Autodesk Fusion 360 part; units mm, degrees
note: some values were not read from the file. Chosen so that the rebuilt part matches the saved one: which face or edge a step refers to; which pieces of a blend or face edit are solid. Set by a fixed rule: which sketch regions a step uses.
(part 2 of 3)
extrude "Extrude11" cut sketch "Blueprint" along normal blind 2 contours A6 picked at (-1.581142, 47.433122) bodies 1
extrude "Extrude12" add sketch "Blueprint" along normal blind 19 separate body contours L20 L21 L22 L23 A16 A57 | L22 A16 | L22 A56 A57 | L22 A55 A56 | L22 A55 | L3 L7 L24 L26 L27 | L1 A25 picked at (4.033973, -37.441718) picked at (-0.443425, -18.400909) picked at (16, -19.512661) picked at (15.901332, -18.893876) picked at (15.699495, -18.321998) picked at (-6.166027, -29.108385) picked at (17.824648, -25.908449) makes body 3
sketch "Sketch4" plane through (0, 19, 0) normal (0, 1, 0) x (-1, 0, 0)
  line L0 (5.49936, 34.775052) -> (5.49936, 22.275052)
  line L1 (5.49936, 22.275052) -> (-17.60064, 22.275052)
  line L2 (-17.60064, 22.275052) -> (-17.60064, 34.775052)
  line L3 (-17.60064, 34.775052) -> (5.49936, 34.775052)
  line L4 (9.49936, 18.275052) -> (9.49936, 38.775052)
  line L5 (9.49936, 38.775052) -> (-21.60064, 38.775052)
  line L6 (-21.60064, 38.775052) -> (-21.60064, 18.275052)
  line L7 (-21.60064, 18.275052) -> (9.49936, 18.275052)
  line L8 (3.49936, 26.775052) -> (7.49936, 26.775052)
  line L9 (7.49936, 26.775052) -> (7.49936, 30.275052)
  line L10 (7.49936, 30.275052) -> (3.49936, 30.275052)
  line L11 (3.49936, 30.275052) -> (3.49936, 26.775052)
  line L12 (3.49936, 26.775052) -> (7.49936, 30.275052) construction
  line L13 (7.49936, 26.775052) -> (3.49936, 30.275052) construction
  point P0 (5.49936, 28.525052)
  dimension "d49" = 4
  dimension "d50" = 3.5
  constraint horizontal L8
  constraint perpendicular L8 L9
  constraint parallel L8 L10
  constraint parallel L9 L11
extrude "Extrude13" cut sketch "Sketch4" against normal blind 17 contours L0 L8 L9 L10 picked at (6.166027, 29.108385) bodies 3
sketch "Sketch5" plane through (-9.49936, 0, 0) normal (-1, 0, 0) x (0, -1, 0)
  line L0 (0, 18.275052) -> (0, 38.775052)
  line L1 (0, 38.775052) -> (-19, 38.775052)
  line L2 (-19, 38.775052) -> (-19, 18.275052)
  line L3 (-19, 18.275052) -> (0, 18.275052)
  line L4 (-2, 25) -> (-15.110279, 25)
  line L5 (-15.110279, 25) -> (-15.110279, 32.050103)
  line L6 (-15.110279, 32.050103) -> (-2, 32.050103)
  line L7 (-2, 32.050103) -> (-2, 25)
  line L8 (-2, 25) -> (-15.110279, 32.050103) construction
  line L9 (-15.110279, 25) -> (-2, 32.050103) construction
  point P0 (-8.555139, 28.525052)
  constraint horizontal L4
  constraint perpendicular L4 L5
  constraint parallel L4 L6
  constraint parallel L5 L7
extrude "Extrude14" cut sketch "Sketch5" against normal blind 5 contours L4 L5 L6 L7 picked at (-6.370093, 27.350035) bodies 3
extrude "Extrude15" add sketch "Shell" along normal blind 45 separate body makes body 4
extrude "Extrude16" add sketch "Blueprint" along normal blind 45 separate body contours L9 L10 L11 A5 picked at (-1.233383, 60.560963) makes body 5
extrude "Extrude17" add sketch "Shell" along normal blind 2 separate body contours A0 picked at (6.427646, -1.832679) makes body 6
ref_plane "WorkPlane2" through (6.05064, 26, 28.525052) normal (0, 1, 0) x (0, 0, 1)
box "BoxPrimitive1" cut length 17 width 50 height 12 placed x (0, 0, -1) y (-1, 0, 0) z (0, 1, 0) at (25.050639, 26, 61.525052) bodies 4
extrude "Extrude19" add sketch "Blueprint" along normal blind 45 separate body contours A7 | A13 | A23 picked at (-25.103811, -35.273245) picked at (-26.11169, -34.534513) picked at (-29.306987, -35.12917) makes body 7
extrude "Extrude20" add sketch "Blueprint" along normal blind 45 separate body contours A8 | A14 | A22 picked at (-25.103811, 34.726755) picked at (-26.063404, 34.821149) picked at (-29.306987, 34.87083) makes body 8
extrude "Extrude21" add sketch "Blueprint" along normal blind 45 separate body contours A9 | A15 | A21 picked at (25.426628, 33.642904) picked at (29.802492, 35.730779) picked at (27.55602, 33.763856) makes body 9
sketch "Sketch7" plane through (0, 26, 0) normal (0, 1, 0) x (-1, 0, 0)
  arc A0 (24.949361, 47.984679) -> (-25.050639, 47.931884) centre (0, 0) ccw
  line L0 (24.949361, 47.984679) -> (24.949361, 50.228104)
  arc A1 (24.949361, 50.228104) -> (-25.050639, 50.17767) centre (0, 0) ccw
  line L1 (-25.050639, 50.17767) -> (-25.050639, 47.931884)
  circle A2 centre (-19.009017, 51.46438) radius 0.8
  circle A3 centre (-12.981322, 53.323346) radius 0.8
  circle A4 centre (-7.269836, 54.399657) radius 0.8
  circle A5 centre (-1.067304, 54.883088) radius 0.8
  circle A6 centre (4.965873, 54.658118) radius 0.8
  circle A7 centre (10.837016, 53.802717) radius 0.8
  circle A8 centre (16.195064, 52.439423) radius 0.8
  circle A9 centre (21.159709, 50.6403) radius 0.8
  dimension "d80" = 1.6
  dimension "d81" = 1.6
  dimension "d82" = 1.6
  dimension "d83" = 1.6
  dimension "d84" = 1.6
  dimension "d85" = 1.6
  dimension "d86" = 1.6
  dimension "d87" = 1.6
  measures "d80" diameter of A2
  measures "d81" diameter of A3
  measures "d82" diameter of A4
  measures "d83" diameter of A5
  measures "d84" diameter of A6
  measures "d85" diameter of A7
  measures "d86" diameter of A8
  measures "d87" diameter of A9
extrude "Extrude22" add sketch "Sketch7" along normal blind 12 contours A0 A2 picked at (-18.916947, 51.228603) bodies 4
extrude "Extrude23" add sketch "Sketch7" along normal blind 12 contours A0 A3 picked at (-13.069534, 53.575351) bodies 4
extrude "Extrude24" add sketch "Sketch7" along normal blind 12 contours A4 picked at (-6.832624, 54.634154) bodies 4
extrude "Extrude25" add sketch "Sketch7" along normal blind 12 contours A5 picked at (-0.753146, 55.064467) bodies 4
extrude "Extrude26" add sketch "Sketch7" along normal blind 12 contours A6 picked at (5.19146, 54.520452) bodies 4
extrude "Extrude27" add sketch "Sketch7" along normal blind 12 contours A7 picked at (11.203399, 54.016143) bodies 4
extrude "Extrude28" add sketch "Sketch7" along normal blind 12 contours A8 picked at (15.936855, 52.760909) bodies 4
extrude "Extrude29" add sketch "Sketch7" along normal blind 12 contours A9 picked at (21.418616, 50.832786) bodies 4
delete_face "DeleteFace1" 2 faces at (-21.958832, 34, 50.602854) (-20.364995, 34, 50.732108) on bodies 4
delete_face "DeleteFace2" 1 faces at (-15.399192, 34, 52.520588) on bodies 4
delete_face "DeleteFace3" 1 faces at (-11.633153, 34, 53.724196) on bodies 4
delete_face "DeleteFace4" 1 faces at (-4.169017, 34, 54.587261) on bodies 4
delete_face "DeleteFace5" 1 faces at (1.769881, 34, 54.500485) on bodies 4
delete_face "DeleteFace6" 1 faces at (8.044162, 34, 54.600699) on bodies 4
delete_face "DeleteFace7" 1 faces at (13.706571, 30, 52.985687) on bodies 4
delete_face "DeleteFace8" 1 faces at (19.672072, 34, 51.911994) on bodies 4
extrude "Extrude30" cut sketch "Blueprint" along normal blind 2 contours A2 | A10 | A11 | A24 picked at (28.037278, -34.616147) picked at (26.387387, -34.993527) picked at (26.938574, -33.213382) picked at (27.869684, -36.306977) bodies 6
extrude "Extrude31" add sketch "Blueprint" along normal blind 40 separate body contours A12 picked at (26.253933, -32.672943) makes body 10
extrude "Extrude32" add 1 faces at (-42.36532, 0, -35.508369) along direction (0, 1, 0) blind 3 from surface at 45 separate body on bodies 4 makes body 11
extrude "Extrude33" add 1 faces at (-1.233383, 45, -60.560963) along direction (0, 1, 0) blind 5 separate body on bodies 5 makes body 12
extrude "Extrude34" add 1 faces at (-42.36532, 0, -35.508369) along direction (0, 1, 0) blind 5 from surface at 45 separate body on bodies 4 makes body 13
extrude "Extrude35" add sketch "Blueprint" against normal blind 2 from surface at 50 separate body contours A0 L454 | A0 L40 L46 A46 L497 | A0 L40 L46 L454 | A0 A46 L497 L498 | A0 L40 L46 A46 L498 | A0 L32 L40 L46 A46 | A0 L32 L40 L46 | A16 L40 L46 A46 L497 | A16 A46 L497 L498 L499 | A0 L32 L40 L46 A46 | A16 L40 L46 A46 L498 L499 | L32 A16 L40 L46 A46 | L30 L31 L33 A16 L40 L46 A33 L423 L428 L429 L437 L440 L441 L449 A43 L455 L456 L457 L490 L491 L494 L495 A49 | A0 L32 L38 | A0 L32 L38 A46 | L32 A16 L40 L46 A46 | A0 L32 L38 A46 | L32 A16 L40 L43 L46 L49 L459 L462 L479 L480 L481 L484 L485 L489 L490 | A0 L38 L48 | A0 L38 L48 A46 | L32 L38 A16 A46 | L32 A16 L40 L41 L46 L47 L397 L400 L401 L407 L408 L411 L415 L416 L423 | A0 L38 L48 A46 | L32 L38 A16 A46 | L33 L40 L43 L46 L49 L489 L490 L491 | L40 L43 L46 L49 L489 L490 | A0 L42 L48 | A0 L42 L48 A46 | L38 A16 L48 A46 | L32 L38 A16 L397 | L40 L41 L46 L47 L416 L423 | L31 L40 L41 L46 L47 L416 L423 L428 | A0 L42 L48 A46 | L38 A16 L48 A46 | L32 L38 A16 L462 | A0 L42 | A0 L42 A46 | A16 L42 L48 A46 | L38 A16 L48 L397 | L32 L38 L41 L47 L397 | L32 L41 L47 L397 L400 | A16 L42 L48 A46 | L38 A16 L48 L462 | L32 L43 L49 L459 L462 | L32 L38 L43 L49 L462 | L33 L43 L49 L481 L489 | L33 L39 L345 L346 L347 L489 L491 | L33 L39 L455 L491 | L22 A16 L42 A46 | A16 L42 L48 L397 | L38 L41 L47 L48 L397 | L31 L32 L37 L38 L41 L47 L396 L399 L400 | L31 L32 L41 L47 L400 | L31 L41 L47 L415 L416 | L31 L37 L428 L429 | L31 L37 L416 L419 L420 L427 L428 | A16 L42 L48 L462 | L38 L43 L48 L49 L462 | L32 L33 L43 L49 L459 | L32 L33 L38 L39 L43 L49 L342 L343 L459 | L33 L43 L49 L481 L484 | L43 L49 L479 L480 L481 L484 L485 | L33 L39 L481 L489 | L33 L455 L456 L457 | L33 L39 L320 L321 L322 L455 L457 | L39 L315 L347 L491 | L39 L315 L455 L491 | L41 L42 L48 L397 | L37 L38 L41 L42 L47 L389 L390 L391 L393 L396 L397 L399 L400 | L31 L41 L47 L400 L401 | L41 L47 L401 L407 L408 L411 L415 | L31 L41 L47 L401 L415 | L31 L37 L415 L416 | L31 L37 L429 L431 L436 L439 L440 | L31 L429 L437 L440 | L37 L416 L418 L419 L425 L427 L428 | L42 L43 L48 L462 | L38 L42 L43 L49 L315 L341 L342 L461 L462 | L33 L43 L49 L459 L484 | L33 L39 L324 L325 L326 L481 L484 | L39 L315 L481 L489 | L39 L315 L345 L489 | L33 L39 L457 L494 | L39 L315 L320 L455 | L39 L220 L313 L315 L347 | L39 L219 L220 L265 L281 L287 L313 L345 L346 L347 | L315 L345 L347 L348 L489 L491 L492 | L20 L21 L22 L23 A16 A57 | L22 A16 | L37 L38 L391 L392 L393 L394 L395 L396 L398 L399 | L37 L38 L395 L396 L398 L399 | L31 L37 L400 L401 | L31 L37 L401 L404 L406 L414 L415 | L31 L37 L440 L441 | L37 L429 L430 L431 L432 L439 L440 | L37 L419 L420 L421 L422 L426 L427 | L37 L419 L422 L424 L425 L426 L427 | L38 L39 L227 L247 L251 L295 L342 L343 | L38 L227 L249 L251 L303 L315 L341 L342 | L33 L39 L459 L484 | L39 L315 L326 L481 | L39 L265 L281 L315 L345 | L30 L33 L494 L495 | L30 L33 L36 L39 L349 L350 L494 L495 | L39 L315 L322 L457 | L39 L315 L457 L494 | L39 L218 L222 L228 L284 L293 L298 L320 L321 L322 | L39 L218 L284 L315 L320 | L315 L320 L322 L323 L455 L457 L458 | L39 L220 L265 L281 L313 L315 | L39 L219 L220 L265 L281 L287 L313 | L220 L265 L266 L273 L281 L313 L315 L345 L347 L348 | L37 L38 L392 L394 L395 L398 | L37 L38 L395 L398 | L37 L401 L402 L403 L404 L412 L414 L415 L417 | L30 L31 L36 L37 L441 L443 L448 L449 | L30 L31 L441 L449 | L37 L431 L432 L433 L434 L438 L439 | L37 L431 L433 L435 L436 L438 L439 | L37 L421 L422 L426 | L37 L422 L424 L426 | L22 A56 A57 | L22 A56 A57 | L38 L39 L227 L247 L251 L295 | L38 L39 L227 L247 L249 L251 L295 L303 L315 | L39 L315 L343 L459 | L39 L315 L459 L484 | L39 L315 L324 L484 | L39 L271 L314 L315 L326 | L39 L216 L231 L252 L267 L271 L314 L324 L325 L326 | L315 L324 L326 L327 L478 L481 L482 L483 L484 | L39 L315 L349 L494 | L39 L222 L228 L315 L322 | L39 L218 L222 L228 L284 L293 L298 | L39 L218 L222 L228 L284 L315 | L218 L222 L228 L237 L240 L284 L315 L320 L322 L323 | L220 L265 L266 L273 L281 L313 L315 | L37 L404 L405 L406 L409 L413 L414 | L37 L403 L404 L409 L410 L413 L414 | L36 L37 L441 L442 L443 L444 L448 L449 L451 L452 | L37 L433 L434 L438 | L37 L433 L435 L438 | L22 A55 A56 | L22 A55 A56 | L315 L341 L343 L344 L459 L460 L461 | L236 L242 L247 L249 L295 L303 L315 L341 L343 L344 | L39 L247 L295 L315 L343 | L39 L231 L252 L315 L324 | L39 L231 L252 L271 L314 L315 | L39 L216 L231 L252 L267 L271 L314 | L231 L252 L268 L271 L275 L314 L315 L324 L326 L327 | L30 L36 A33 L495 | L36 L39 L229 L254 L299 L309 L349 L350 | L39 L229 L254 L315 L349 | L315 L349 L351 L352 L493 L494 L496 | L218 L222 L228 L237 L240 L284 L315 | L37 L405 L409 L413 | L37 L409 L410 L413 | L30 L36 L449 A43 | L36 L37 L443 L444 L445 L446 L447 L448 L450 L451 | L36 L37 L443 L446 L447 L448 | L22 A55 | L22 A55 | L236 L242 L247 L249 L295 L303 L315 | L231 L252 L268 L271 L275 L314 L315 | L30 A32 A33 | L30 L36 A32 A33 | L36 L315 L350 L351 L495 L496 | L36 L39 L229 L254 L299 L309 | L36 L39 L223 L229 L254 L292 L299 L309 L315 | L223 L229 L234 L241 L254 L292 L315 L349 L351 L352 | L30 L36 A43 A44 | L30 A43 A44 | L36 L37 L445 L446 L447 L450 | L36 L37 L446 L447 | L30 A31 A32 | L30 L36 A31 A32 | L30 L36 A32 A33 | L30 L36 A33 A49 | L36 A32 A33 | L36 L223 L292 L299 L309 L315 L350 L351 | L223 L229 L234 L241 L254 L292 L315 | L30 L36 A44 A45 | L30 A44 A45 | L36 A43 A44 | L30 L36 A43 A49 | L30 L36 A43 A44 | L30 A31 | L30 L36 A31 | L30 L36 A31 A32 | L36 A31 A32 | L30 A49 A51 | L30 L36 A49 A51 | L30 L36 A45 | L30 A45 | L36 A44 A45 | L30 L36 A44 A45 | L30 L36 A49 A51 | L36 A31 | L30 A50 A51 | L30 L36 A50 A51 | L36 A49 A51 | L36 A45 | L30 L36 A50 A51 | L30 A50 | L30 L36 A50 | L36 A50 A51 | L36 A50 | L0 L2 L3 L4 L5 L6 L7 L24 L25 L26 | L0 L1 L2 L5 A25 | L3 L7 L24 L26 L27 | L3 L7 L24 L25 L26 | L1 A25 | L1 A25 | L8 L9 L11 A5 | L8 L9 L11 L14 L15 L17 A5 | L14 L15 L17 A5 | A1 | A2 | A3 | A4 | A6 | A7 | A8 | A9 | A10 | A11 | A12 | A13 | A14 | A15 | A17 | A18 | A19 | A21 | A22 | A23 | A24 | L235 L260 L270 L286 L288 L301 L315 L328 L329 L331 | L235 L260 L270 L286 L288 L301 L315 | L246 L259 L260 L286 L288 L301 L315 | L246 L259 L260 L286 L288 L301 L315 L329 L330 L331 | L315 L329 L330 L331 L471 L472 L473 | L315 L328 L329 L331 L471 L473 L474 | L238 L243 L244 L248 L264 L307 L315 L332 L334 L335 | L238 L243 L244 L248 L264 L307 L315 | L244 L248 L264 L279 L300 L307 L315 | L244 L248 L264 L279 L300 L307 L315 L332 L333 L334 | L315 L332 L333 L334 L464 L465 L466 | L315 L332 L334 L335 L463 L464 L466 | L239 L245 L272 L278 L290 L297 L315 L336 L338 L339 | L239 L245 L272 L278 L290 L297 L315 | L245 L261 L278 L289 L290 L297 L315 | L245 L261 L278 L289 L290 L297 L315 L336 L337 L338 | L315 L336 L337 L338 L467 L468 L470 | L315 L336 L338 L339 L468 L469 L470 | A26 | A27 | A28 | A29 | A30 | A34 | A35 | A36 | A37 | A38 | A39 | L353 L354 L355 L356 | L357 L360 L362 L363 | L358 L359 L361 L364 | L365 L366 L367 L376 | L368 L371 L373 L375 | L369 L370 L372 L374 | L377 L378 L379 L388 | L380 L383 L385 L387 | L381 L382 L384 L386 | A40 | A41 | A42 | A52 | A53 | A54 picked at (-0.080266, 16.579553) picked at (9.705176, 15.068275) picked at (-3, 10.157626) picked at (-7.671277, 16.192817) picked at (-9.705176, 15.068275) picked at (16.610892, 6.696031) picked at (5.417667, 1.4) picked at (10.29341, 15.063896) picked at (8.168486, 16.306197) picked at (-16.588449, 6.769971) picked at (-10.29341, 15.063896) picked at (16.955543, 6.695503) picked at (-18.919314, 15.014678) picked at (-5.900918, -1.983333) picked at (-17.768839, -2.539148) picked at (-16.933326, 6.769391) picked at (17.768839, -2.539148) picked at (22.633332, 0.538942) picked at (-5.882271, -2.766667) picked at (-17.703996, -2.961152) picked at (-18.088769, -2.539143) picked at (-22.551552, 3.200808) picked at (17.703996, -2.961152) picked at (18.088769, -2.539143) picked at (24.886666, 10.733333) picked at (24.733332, 6.85) picked at (5.683555, -5.514289) picked at (-16.506733, -7.014289) picked at (-18.061761, -2.727855) picked at (-22.598153, -2.094669) picked at (-24.866667, 6.85) picked at (-24.886667, 10.733333) picked at (16.506733, -7.014289) picked at (18.061761, -2.727855) picked at (22.59815, -2.094669) picked at (-1.266033, -11.46973) picked at (15.487236, -8.996433) picked at (-16.85228, -7.014027) picked at (-22.570428, -2.766667) picked at (-24.866667, -1.983333) picked at (-24.733335, -1.583333) picked at (16.85228, -7.014027) picked at (22.570425, -2.766667) picked at (24.733332, -1.516667) picked at (24.733332, -1.983333) picked at (25.04, 5.483333) picked at (25.489999, 12.1) picked at (25.393333, 12.416666) picked at (-3.872417, -17.820116) picked at (-22.447225, -5.011798) picked at (-24.866667, -2.766667) picked at (-25.490001, -1.766667) picked at (-25.02, -1.583333) picked at (-25.02, 5.483333) picked at (-25.393333, 12.383333) picked at (-25.490001, 12.1) picked at (22.447222, -5.011798) picked at (24.866666, -2.883333) picked at (25.04, -1.583333) picked at (25.489999, -1.766667) picked at (25.02, 3.183333) picked at (24.866666, 2.355609) picked at (25.726667, 5.483333) picked at (24.906666, 14.716666) picked at (25.489999, 12.7) picked at (27.353333, 11.85) picked at (27.353333, 12.383333) picked at (-24.866667, -4.5) picked at (-28.883336, -8) picked at (-25.02, -1.416667) picked at (-24.866667, 1.744392) picked at (-25.04, 3.183333) picked at (-25.726667, 5.516666) picked at (-25.490001, 19) picked at (-24.906667, 16.983333) picked at (-31.150002, 9.833333) picked at (24.733332, -4.5) picked at (25.983332, -8) picked at (25.02, -1.383334) picked at (25.489999, -1.1) picked at (27.353333, 5.483333) picked at (27.353333, 5.8) picked at (25.393333, 19.316666) picked at (27.353333, 12.7) picked at (27.353333, 11.5) picked at (25.399998, 8.116666) picked at (31.149998, 8.066666) picked at (4.033973, -37.441718) picked at (-0.443425, -18.400909) picked at (-27.166669, -7.45) picked at (-25.636668, -2.25) picked at (-25.726667, -1.383334) picked at (-25.490001, -1.1) picked at (-25.393333, 19.283333) picked at (-31.150002, 14.966666) picked at (-25.400002, 8.116666) picked at (-30.600002, 8.116666) picked at (25.636665, -2.25) picked at (25.399998, -5.833333) picked at (25.393333, -1.383334) picked at (27.353333, 4.95) picked at (27.353333, 6.35) picked at (24.906666, 20.116667) picked at (25.489999, 19.6) picked at (27.353333, 18.75) picked at (27.353333, 19.283333) picked at (25.399998, 16.683333) picked at (27.353333, 13.25) picked at (31.149998, 14.966666) picked at (27.353333, 8.116666) picked at (25.873333, 8.116666) picked at (30.599998, 8.116666) picked at (-27.353335, -5.783333) picked at (-25.873334, -2.45) picked at (-30.900002, 2.355609) picked at (-25.490001, 19.6) picked at (-24.906667, 20.883333) picked at (-30.600002, 16.683333) picked at (-25.400002, 15.016666) picked at (-25.873334, 9.783333) picked at (-29.020002, 9.783333) picked at (14.100388, -18.043793) picked at (16, -19.512661) picked at (25.686665, -2.45) picked at (26.519999, -5.783333) picked at (27.353333, -1.95) picked at (27.353333, -1.416667) picked at (27.353333, -1.1) picked at (27.353333, 4.6) picked at (25.399998, 1.216666) picked at (30.899998, 1.744392) picked at (27.353333, 19.6) picked at (27.353333, 18.4) picked at (25.873333, 15.016666) picked at (27.353333, 15.016666) picked at (30.599998, 15.016666) picked at (28.833332, 9.783333) picked at (-25.400002, 1.216666) picked at (-30.600002, 1.216666) picked at (-31.150002, 21.866666) picked at (-27.540001, 15.016666) picked at (-25.873334, 16.683333) picked at (14.799711, -18.162342) picked at (15.901332, -18.893876) picked at (31.149998, -5.733334) picked at (30.599998, -4.016667) picked at (27.353333, -2.3) picked at (27.353333, -0.55) picked at (27.353333, 1.216666) picked at (25.686665, 2.883333) picked at (30.599998, 2.883333) picked at (22.473627, 22.229735) picked at (25.399998, 21) picked at (27.353333, 20.15) picked at (31.149998, 21.866666) picked at (28.833332, 16.683333) picked at (-25.873334, 2.883333) picked at (-29.020002, 2.883333) picked at (-22.806963, 22.229735) picked at (-27.166669, 25.35) picked at (-25.400002, 21) picked at (15.900371, -17.570903) picked at (15.699495, -18.321998) picked at (28.833333, -4.016667) picked at (28.833333, 2.883333) picked at (14.739817, 21.245372) picked at (17.917968, 22.326792) picked at (24.849998, 24.733333) picked at (25.873333, 21.05) picked at (27.353333, 22.716667) picked at (30.599998, 21.916666) picked at (-18.917967, 22.326792) picked at (-18.260183, 21.245372) picked at (-29.020002, 22.716667) picked at (-25.873334, 21.85) picked at (15.401746, 21.543061) picked at (16.918149, 21.76373) picked at (14.082033, 22.326792) picked at (6.082593, 22.476137) picked at (14.039145, 22.826574) picked at (25.399998, 24.433333) picked at (28.833332, 23.583333) picked at (-17.918148, 21.76373) picked at (-16.401745, 21.543061) picked at (-18.960855, 22.826574) picked at (-6.415925, 22.476137) picked at (-15.082032, 22.326792) picked at (16.144253, 21.625767) picked at (15.793173, 22.25812) picked at (15.081852, 21.76373) picked at (14.653406, 22.779056) picked at (-1.260183, 21.245372) picked at (1.917968, 22.326792) picked at (-16.76103, 22.289882) picked at (-16.855747, 21.625767) picked at (-18.346594, 22.779056) picked at (-16.081851, 21.76373) picked at (-1.917967, 22.326792) picked at (16.399841, 22.897923) picked at (-0.598254, 21.543061) picked at (0.918149, 21.76373) picked at (-1.960855, 22.826574) picked at (-16.838019, 23.067226) picked at (-0.918148, 21.76373) picked at (-0.144252, 21.625767) picked at (0.269322, 21.884696) picked at (-1.346594, 22.779056) picked at (0.161981, 23.067226) picked at (-1.166027, -27.941718) picked at (4.61622, -27.751627) picked at (-6.166027, -29.108385) picked at (-4.832694, -27.941718) picked at (17.274712, -27.041797) picked at (17.824648, -25.908449) picked at (-19.500414, 45.97393) picked at (-0.092673, 33.048676) picked at (1.364052, -47.916694) picked at (-28.447805, -34.584499) picked at (28.037278, -34.616147) picked at (27.665869, 35.49322) picked at (-28.447805, 35.415501) picked at (-1.581142, 47.433122) picked at (-25.103811, -35.273245) picked at (-25.103811, 34.726755) picked at (25.426628, 33.642904) picked at (26.387387, -34.993527) picked at (26.938574, -33.213382) picked at (26.253933, -32.672943) picked at (-26.11169, -34.534513) picked at (-26.063404, 34.821149) picked at (29.802492, 35.730779) picked at (38.740213, -25.999966) picked at (39.611389, -23.686242) picked at (37.680599, -25.819207) picked at (27.55602, 33.763856) picked at (-29.306987, 34.87083) picked at (-29.306987, -35.12917) picked at (27.869684, -36.306977) picked at (30.599998, -10.916667) picked at (28.833333, -10.916667) picked at (27.166666, -12.583334) picked at (25.399998, -12.583334) picked at (24.849998, -12.633334) picked at (31.149998, -12.633334) picked at (30.599998, -17.816667) picked at (28.833333, -17.816667) picked at (27.166666, -19.483334) picked at (25.399998, -19.483334) picked at (24.849998, -17.766667) picked at (31.149998, -19.533334) picked at (30.599998, -24.716667) picked at (28.833333, -24.716667) picked at (27.166666, -26.383334) picked at (25.399998, -26.383334) picked at (24.849998, -24.666667) picked at (31.149998, -26.433334) picked at (16.330409, -25.375998) picked at (17.340134, -25.681655) picked at (39.344267, 22.860514) picked at (39.611389, 24.613758) picked at (37.680599, 22.480793) picked at (-39.655733, -25.439486) picked at (-41.319401, -25.819207) picked at (-39.388611, -23.686242) picked at (-15.04171, -25.661782) picked at (-15.655212, -25.619554) picked at (-16.643107, -25.607971) picked at (-31.150002, -24.666667) picked at (-25.400002, -26.383334) picked at (-28.833336, -24.716667) picked at (-31.150002, -17.766667) picked at (-27.166669, -21.25) picked at (-27.166669, -19.483334) picked at (-28.883336, -14.9) picked at (-25.400002, -10.916667) picked at (-27.166669, -12.583334) picked at (-41.319401, 22.480793) picked at (-39.655733, 22.860514) picked at (-39.388611, 24.613758) picked at (-16.643107, -17.607971) picked at (-15.655212, -17.619554) picked at (-15.046922, -17.731335) makes body 14
sketch "Sketch8" plane through (0, 48, 0) normal (0, 1, 0) x (-1, 0, 0)
  circle A0 centre (0, 0) radius 53.966054
  circle A1 centre (-28, 35.000001) radius 1.25
  circle A2 centre (-28, 35.000001) radius 1.75
  circle A3 centre (-28, 35.000001) radius 2.236068
  circle A4 centre (0, 0) radius 54.966054
  circle A5 centre (-28, 35.000001) radius 3.4
  circle A6 centre (-28, 35.000001) radius 4.9
  circle A7 centre (0, 0) radius 18.05
  circle A8 centre (0, 0) radius 18.7
  line L0 (-9, -15.472879) -> (9, -15.472879)
  line L1 (9.294757, -15.472879) -> (10.501428, -15.472879)
  line L2 (9, -15.472879) -> (10.8, -15.472879)
  line L3 (-9, -15.472879) -> (-11.1, -15.472879)
  circle A9 centre (-16, 17.550001) radius 2.25
  circle A10 centre (-16, 17.550001) radius 1.4
  circle A11 centre (-16, 17.550001) radius 1.25
  circle A12 centre (-16, 25.550001) radius 1.25
  circle A13 centre (-16, 25.550001) radius 1.4
  circle A14 centre (-16, 25.550001) radius 2.25
  circle A15 centre (17, 25.550001) radius 2.25
  circle A16 centre (17, 25.550001) radius 1.25
  circle A17 centre (17, 25.550001) radius 1.4
  circle A18 centre (17, 17.550001) radius 2.25
  circle A19 centre (17, 17.550001) radius 1.4
  circle A20 centre (17, 17.550001) radius 1.25
  circle A21 centre (40, 25.550001) radius 2.25
  circle A22 centre (40, 25.550001) radius 1.25
  circle A23 centre (40, 25.550001) radius 1.4
  circle A24 centre (40, -22.749999) radius 2.25
  circle A25 centre (40, -22.749999) radius 1.4
  circle A26 centre (40, -22.749999) radius 1.25
  circle A27 centre (17, -22.749999) radius 2.25
  circle A28 centre (17, -22.749999) radius 1.4
  circle A29 centre (17, -22.749999) radius 1.25
  circle A30 centre (0, -22.749999) radius 2.25
  circle A31 centre (0, -22.749999) radius 1.4
  circle A32 centre (0, -22.749999) radius 1.25
  circle A33 centre (-16, -22.749999) radius 2.25
  circle A34 centre (-16, -22.749999) radius 1.4
  circle A35 centre (-16, -22.749999) radius 1.25
  circle A36 centre (-39, -22.749999) radius 2.25
  circle A37 centre (-39, -22.749999) radius 1.4
  circle A38 centre (-39, -22.749999) radius 1.25
  circle A39 centre (-39, 25.550001) radius 2.25
  circle A40 centre (-39, 25.550001) radius 1.4
  circle A41 centre (-39, 25.550001) radius 1.25
  line L4 (-30.649998, 28.2) -> (-25.349998, 28.2)
  line L5 (-25.349998, 28.2) -> (-25.349998, 22.9)
  line L6 (-25.349998, 22.9) -> (-30.649998, 22.9)
  line L7 (-30.649998, 22.9) -> (-30.649998, 28.2)
  line L8 (-31.399998, 28.95) -> (-24.599998, 28.95)
  line L9 (-24.599998, 28.95) -> (-24.599998, 22.15)
  line L10 (-24.599998, 22.15) -> (-31.399998, 22.15)
  line L11 (-31.399998, 22.15) -> (-31.399998, 28.95)
  line L12 (-31.399998, 22.05) -> (-24.599998, 22.05)
  line L13 (-24.599998, 22.05) -> (-24.599998, 15.25)
  line L14 (-25.349998, 21.3) -> (-25.349998, 16)
  line L15 (-30.649998, 21.3) -> (-25.349998, 21.3)
  line L16 (-30.649998, 16) -> (-30.649998, 21.3)
  line L17 (-31.399998, 15.25) -> (-31.399998, 22.05)
  line L18 (-25.349998, 16) -> (-30.649998, 16)
  line L19 (-24.599998, 15.25) -> (-31.399998, 15.25)
  line L20 (-24.599998, 15.15) -> (-24.599998, 8.35)
  line L21 (-31.399998, 15.15) -> (-24.599998, 15.15)
  line L22 (-22, 15.200001) -> (-34, 15.200001)
  line L23 (-31.399998, 8.35) -> (-31.399998, 15.15)
  line L24 (-25.349998, 14.4) -> (-25.349998, 9.1)
  line L25 (-30.649998, 14.4) -> (-25.349998, 14.4)
  line L26 (-30.649998, 9.1) -> (-30.649998, 14.4)
  line L27 (-25.349998, 9.1) -> (-30.649998, 9.1)
  line L28 (-24.599998, 8.35) -> (-31.399998, 8.35)
  line L29 (-31.399998, 8.25) -> (-24.599998, 8.25)
  line L30 (-24.599998, 8.25) -> (-24.599998, 1.45)
  line L31 (-30.649998, 7.5) -> (-25.349998, 7.5)
  line L32 (-30.649998, 2.2) -> (-30.649998, 7.5)
  line L33 (-31.399998, 1.45) -> (-31.399998, 8.25)
  line L34 (-25.349998, 7.5) -> (-25.349998, 2.2)
  line L35 (-25.349998, 2.2) -> (-30.649998, 2.2)
  line L36 (-24.599998, 1.45) -> (-31.399998, 1.45)
  line L37 (-31.399998, 1.35) -> (-24.599998, 1.35)
  line L38 (-24.599998, 1.35) -> (-24.599998, -2.966827)
  line L39 (-30.649998, 0.6) -> (-25.349998, 0.6)
  line L40 (-25.349998, 0.6) -> (-25.349998, -4.7)
  line L41 (-30.649998, -4.7) -> (-30.649998, 0.6)
  line L42 (-31.399998, -1.133176) -> (-31.399998, 0.943173)
  line L43 (-31.399998, 0.943173) -> (-31.399998, 1.35)
  line L44 (-31.399998, -5.45) -> (-31.399998, -1.133176)
  line L45 (-24.599998, -2.966827) -> (-24.599998, -5.043176)
  line L46 (-24.599998, -5.043176) -> (-24.599998, -5.45)
  line L47 (-24.599998, -5.45) -> (-31.399998, -5.45)
  line L48 (-24.599998, -5.55) -> (-24.599998, -12.35)
  line L49 (-31.399998, -5.55) -> (-24.599998, -5.55)
  line L50 (-30.649998, -6.3) -> (-25.349998, -6.3)
  line L51 (-30.649998, -11.6) -> (-30.649998, -6.3)
  line L52 (-25.349998, -6.3) -> (-25.349998, -11.6)
  line L53 (-31.399998, -12.35) -> (-31.399998, -5.55)
  line L54 (-25.349998, -11.6) -> (-30.649998, -11.6)
  line L55 (-24.599998, -12.45) -> (-24.599998, -19.25)
  line L56 (-30.649998, -13.2) -> (-25.349998, -13.2)
  line L57 (-24.599998, -12.35) -> (-31.399998, -12.35)
  line L58 (-31.399998, -12.45) -> (-24.599998, -12.45)
  line L59 (-31.399998, -19.25) -> (-31.399998, -12.45)
  line L60 (-30.649998, -18.5) -> (-30.649998, -13.2)
  line L61 (-25.349998, -13.2) -> (-25.349998, -18.5)
  line L62 (-25.349998, -18.5) -> (-30.649998, -18.5)
  line L63 (-31.399998, -19.35) -> (-24.599998, -19.35)
  line L64 (-24.599998, -19.25) -> (-31.399998, -19.25)
  line L65 (-24.599998, -19.35) -> (-24.599998, -26.15)
  line L66 (-31.399998, -26.15) -> (-31.399998, -19.35)
  line L67 (-30.649998, -20.1) -> (-25.349998, -20.1)
  line L68 (-25.349998, -20.1) -> (-25.349998, -25.4)
  line L69 (-30.649998, -25.4) -> (-30.649998, -20.1)
  line L70 (-25.349998, -25.4) -> (-30.649998, -25.4)
  line L71 (-24.599998, -26.15) -> (-31.399998, -26.15)
  line L72 (-25.349998, -4.7) -> (-30.649998, -4.7)
  line L73 (-30.499998, 0.45) -> (-25.499998, 0.45)
  line L74 (-25.499998, 0.45) -> (-25.499998, -4.55)
  line L75 (-30.499998, -4.55) -> (-30.499998, 0.45)
  line L76 (-25.499998, -4.55) -> (-30.499998, -4.55)
  line L77 (25.350002, 28.2) -> (30.650002, 28.2)
  line L78 (25.350002, 22.9) -> (25.350002, 28.2)
  line L79 (24.600002, 22.15) -> (24.600002, 28.95)
  line L80 (24.600002, 28.95) -> (31.400002, 28.95)
  line L81 (31.400002, 28.95) -> (31.400002, 22.15)
  line L82 (30.650002, 28.2) -> (30.650002, 22.9)
  line L83 (31.400002, 22.15) -> (24.600002, 22.15)
  line L84 (30.650002, 22.9) -> (25.350002, 22.9)
  line L85 (24.600002, 22.05) -> (31.400002, 22.05)
  line L86 (24.600002, 15.25) -> (24.600002, 22.05)
  line L87 (25.350002, 21.3) -> (30.650002, 21.3)
  line L88 (25.350002, 16) -> (25.350002, 21.3)
  line L89 (30.650002, 21.3) -> (30.650002, 16)
  line L90 (31.400002, 22.05) -> (31.400002, 15.25)
  line L91 (30.650002, 16) -> (25.350002, 16)
  line L92 (31.400002, 15.25) -> (24.600002, 15.25)
  line L93 (24.600002, 15.15) -> (31.400002, 15.15)
  line L94 (24.600002, 8.35) -> (24.600002, 15.15)
  line L95 (25.350002, 14.4) -> (30.650002, 14.4)
  line L96 (25.350002, 9.1) -> (25.350002, 14.4)
  line L97 (30.650002, 14.4) -> (30.650002, 9.1)
  line L98 (31.400002, 15.15) -> (31.400002, 8.35)
  line L99 (31.400002, 8.35) -> (24.600002, 8.35)
  line L100 (30.650002, 9.1) -> (25.350002, 9.1)
  line L101 (24.600002, 1.45) -> (24.600002, 8.25)
  line L102 (25.350002, 7.5) -> (30.650002, 7.5)
  line L103 (24.600002, 8.25) -> (31.400002, 8.25)
  line L104 (25.350002, 2.2) -> (25.350002, 7.5)
  line L105 (30.650002, 7.5) -> (30.650002, 2.2)
  line L106 (31.400002, 8.25) -> (31.400002, 1.45)
  line L107 (31.400002, 1.45) -> (24.600002, 1.45)
  line L108 (30.650002, 2.2) -> (25.350002, 2.2)
  line L109 (24.600002, 1.35) -> (31.400002, 1.35)
  line L110 (24.600002, 0.943173) -> (24.600002, 1.35)
  line L111 (24.600002, -1.133176) -> (24.600002, 0.943173)
  line L112 (25.350002, 0.6) -> (30.650002, 0.6)
  line L113 (25.350002, -4.7) -> (25.350002, 0.6)
  line L114 (30.650002, 0.6) -> (30.650002, -4.7)
  line L115 (31.400002, 1.35) -> (31.400002, -2.966827)
  line L116 (24.600002, -5.45) -> (24.600002, -1.133176)
  line L117 (30.650002, -4.7) -> (25.350002, -4.7)
  line L118 (31.400002, -2.966827) -> (31.400002, -5.043176)
  line L119 (31.400002, -5.043176) -> (31.400002, -5.45)
  line L120 (31.400002, -5.45) -> (24.600002, -5.45)
  line L121 (24.600002, -12.35) -> (24.600002, -5.55)
  line L122 (24.600002, -5.55) -> (31.400002, -5.55)
  line L123 (25.350002, -6.3) -> (30.650002, -6.3)
  line L124 (25.350002, -11.6) -> (25.350002, -6.3)
  line L125 (30.650002, -6.3) -> (30.650002, -11.6)
  line L126 (31.400002, -5.55) -> (31.400002, -12.35)
  line L127 (30.650002, -11.6) -> (25.350002, -11.6)
  line L128 (31.400002, -12.35) -> (24.600002, -12.35)
  line L129 (24.600002, -12.45) -> (31.400002, -12.45)
  line L130 (24.600002, -19.25) -> (24.600002, -12.45)
  line L131 (25.350002, -13.2) -> (30.650002, -13.2)
  line L132 (25.350002, -18.5) -> (25.350002, -13.2)
  line L133 (30.650002, -13.2) -> (30.650002, -18.5)
  line L134 (31.400002, -12.45) -> (31.400002, -19.25)
  line L135 (30.650002, -18.5) -> (25.350002, -18.5)
  line L136 (31.400002, -19.25) -> (24.600002, -19.25)
  line L137 (24.600002, -19.35) -> (31.400002, -19.35)
  line L138 (24.600002, -26.15) -> (24.600002, -19.35)
  line L139 (25.350002, -20.1) -> (30.650002, -20.1)
  line L140 (30.650002, -20.1) -> (30.650002, -25.4)
  line L141 (31.400002, -19.35) -> (31.400002, -26.15)
  line L142 (25.350002, -25.4) -> (25.350002, -20.1)
  line L143 (30.650002, -25.4) -> (25.350002, -25.4)
  line L144 (31.400002, -26.15) -> (24.600002, -26.15)
  line L145 (11, 22) -> (21.301271, 22)
  line L146 (21.301271, 22) -> (21.301271, 11.324357)
  line L147 (21.301271, -12.494508) -> (21.301271, -17.258282)
  line L148 (21.301271, -17.258282) -> (18, -17.258282)
  line L149 (45.000001, -25) -> (45.000001, 23)
  line L150 (21.301271, 11.324357) -> (21.301271, -12.494508)
  line L151 (-21.250421, -18.21566) -> (-21.250421, -7.540017)
  line L152 (-10.94915, -18.21566) -> (-21.250421, -18.21566)
  line L153 (-10.94915, -27.21566) -> (-10.94915, -18.21566)
  line L154 (-36.949151, -27.21566) -> (-10.94915, -27.21566)
  arc A42 (-44.949151, -19.21566) -> (-36.949151, -27.21566) centre (-36.949151, -19.21566) ccw
  line L155 (-21.250421, 16.278849) -> (-21.250421, 21.042622)
  line L156 (-21.250421, -7.540017) -> (-21.250421, 16.278849)
  line L157 (-12, 29.5) -> (-42.000001, 29.5)
  line L158 (-44.949151, -19.21566) -> (-44.949151, 24)
  arc A43 (-42.000001, 29.5) -> (-45.000001, 27) centre (-42.000001, 26.45) ccw
  line L159 (-45.000001, 27) -> (-44.949151, 24)
  line L160 (41.392022, 29.5) -> (11, 29.5)
  arc A44 (11, 29.5) -> (11, 22) centre (12.137721, 25.75) ccw
  arc A45 (45.000001, 27) -> (41.392022, 29.5) centre (41.392022, 25.646498) ccw
  line L161 (45.000001, 27) -> (45.000001, 23)
  arc A46 (42.803198, -27.21566) -> (45.000001, -25) centre (42.78426, -25) ccw
  line L162 (18, -17.258282) -> (13, -17.258282)
  line L163 (42.803198, -27.21566) -> (13, -27.21566)
  line L164 (13, -17.258282) -> (13, -27.21566)
  line L165 (20, 21) -> (20, 16.662179)
  arc A47 (17, 13) -> (20, 16.662179) centre (16.525865, 16.44827) ccw
  line L166 (17, 13) -> (8, 13)
  line L167 (8, 13) -> (8, 16.902367)
  line L168 (11, 21) -> (8, 16.902367)
  line L169 (11, 21) -> (20, 21)
  line L170 (-10.754507, 12.683289) -> (-19.754507, 12.683289)
  line L171 (-19.754507, 12.683289) -> (-19.754507, 17.02111)
  arc A48 (-16.754507, 20.683289) -> (-19.754507, 17.02111) centre (-16.280372, 17.235018) ccw
  line L172 (-10.754507, 12.683289) -> (-9, 12.683289)
  line L173 (-9, 12.683289) -> (-9, 16.391766)
  line L174 (-9, 16.391766) -> (-12, 20)
  line L175 (-21.250421, 21.042622) -> (-21.250421, 22)
  line L176 (-21.250421, 22) -> (-12, 22)
  arc A49 (-12, 22) -> (-12, 29.5) centre (-12.833334, 25.75) ccw
  line L177 (-12, 20) -> (-12.568108, 20.683289)
  line L178 (-12.568108, 20.683289) -> (-16.754507, 20.683289)
  line L179 (4, -27) -> (-4, -27)
  line L180 (-4, -27) -> (-10.05, -12.611032)
  line L181 (-10.05, -12.611032) -> (10, -12.611032)
  line L182 (10, -12.611032) -> (4, -27)
  point P0 (-24.599998, 15.25)
  dimension "d122" = 2.5
  dimension "d123" = 3.5
  dimension "d128" = 6.8
  dimension "d129" = 1.5
  constraint concentric A1 A2
  constraint concentric A1 A3
  constraint concentric A1 A5
  constraint perpendicular L145 L146
  constraint vertical L147
  constraint perpendicular L147 L148
  constraint vertical L149
  constraint parallel L147 L150
  constraint perpendicular L153 L154
  constraint perpendicular L152 L153
  constraint perpendicular L151 L152
  constraint tangent L154 A42
  constraint parallel L155 L156
  constraint horizontal L157
  constraint tangent A42 L158
  constraint vertical L158
  constraint tangent L157 A43
  constraint parallel L157 L160
  constraint tangent L160 A45
  constraint parallel L149 L161
  constraint tangent L149 A46
  constraint perpendicular L130 L162
  constraint horizontal L163
  constraint perpendicular L163 L164
  constraint parallel L146 L165
  constraint horizontal L166
  constraint perpendicular L166 L167
  constraint perpendicular L165 L169
  constraint perpendicular L170 L171
  constraint parallel L170 L172
  constraint perpendicular L170 L173
  constraint perpendicular L145 L175
  constraint perpendicular L155 L176
  constraint parallel L174 L177
  constraint horizontal L178
  constraint perpendicular L125 L179
  constraint parallel L3 L181
  measures "d122" diameter of A1
  measures "d123" diameter of A2
  measures "d128" diameter of A5
sketch "Sketch9" plane through (0, 40, 0) normal (0, 1, 0) x (-1, 0, 0)
  circle A0 centre (-28, 35.000001) radius 2.25
  circle A1 centre (-28, 35.000001) radius 3.25
  circle A2 centre (-28, 35.000001) radius 1.3
  dimension "d125" = 2.6
  constraint concentric A0 A2
  measures "d125" diameter of A2
extrude "Extrude36" add sketch "Sketch9" against normal blind 3 separate body contours A0 picked at (-26.075044, 34.888219) makes body 15
extrude "Extrude37" add sketch "Sketch8" against normal blind 8 separate body contours A2 picked at (-26.617059, 34.237513) makes body 16
extrude "Extrude38" add sketch "Sketch8" against normal blind 8 separate body contours A3 | A5 picked at (-29.769358, 36.071876) picked at (-25.008961, 34.719996) makes body 17
extrude "Extrude39" add sketch "Sketch8" against normal blind 16 separate body contours A6 picked at (-23.630902, 34.58765) makes body 18
copy_body "CopyPasteBodies1" bodies 10 15 16 17 18 makes body 19 makes body 20 makes body 21 makes body 22 makes body 23
move_body "Move1" bodies 19 20 21 22 23 to x (1, 0, 0) y (0, 1, 0) z (0, 0, 1) at (-59, 0, 0)
extrude "Extrude40" add sketch "Blueprint" along normal blind 12 separate body contours A0 L32 L38 | A0 L32 L38 A46 | A0 L32 L38 A46 | L32 L38 A16 A46 | L32 L38 A16 A46 | L32 L38 A16 L397 | L32 L38 A16 L462 | L32 L38 L41 L47 L397 | L32 L38 L43 L49 L462 | L33 L39 L345 L346 L347 L489 L491 | L33 L39 L455 L491 | L31 L32 L37 L38 L41 L47 L396 L399 L400 | L31 L37 L428 L429 | L31 L37 L416 L419 L420 L427 L428 | L32 L33 L38 L39 L43 L49 L342 L343 L459 | L33 L39 L481 L489 | L33 L39 L320 L321 L322 L455 L457 | L31 L37 L415 L416 | L31 L37 L429 L431 L436 L439 L440 | L33 L39 L324 L325 L326 L481 L484 | L33 L39 L457 L494 | L39 L219 L220 L265 L281 L287 L313 L345 L346 L347 | L37 L38 L395 L396 L398 L399 | L31 L37 L400 L401 | L31 L37 L401 L404 L406 L414 L415 | L31 L37 L440 L441 | L37 L419 L420 L421 L422 L426 L427 | L38 L39 L227 L247 L251 L295 L342 L343 | L33 L39 L459 L484 | L30 L33 L36 L39 L349 L350 L494 L495 | L39 L218 L222 L228 L284 L293 L298 L320 L321 L322 | L39 L219 L220 L265 L281 L287 L313 | L37 L38 L395 L398 | L30 L31 L36 L37 L441 L443 L448 L449 | L37 L431 L433 L435 L436 L438 L439 | L37 L421 L422 L426 | L38 L39 L227 L247 L251 L295 | L39 L216 L231 L252 L267 L271 L314 L324 L325 L326 | L39 L218 L222 L228 L284 L293 L298 | L37 L404 L405 L406 L409 L413 L414 | L37 L433 L435 L438 | L39 L216 L231 L252 L267 L271 L314 | L30 L36 A33 L495 | L36 L39 L229 L254 L299 L309 L349 L350 | L37 L405 L409 L413 | L30 L36 L449 A43 | L36 L37 L443 L446 L447 L448 | L30 L36 A32 A33 | L36 L39 L229 L254 L299 L309 | L30 L36 A43 A44 | L36 L37 L446 L447 | L30 L36 A31 A32 | L30 L36 A32 A33 | L30 L36 A33 A49 | L30 L36 A44 A45 | L30 L36 A43 A49 | L30 L36 A43 A44 | L30 L36 A31 | L30 L36 A31 A32 | L30 L36 A49 A51 | L30 L36 A45 | L30 L36 A44 A45 | L30 L36 A49 A51 | L30 L36 A50 A51 | L30 L36 A50 A51 | L30 L36 A50 picked at (-5.900918, -1.983333) picked at (-17.768839, -2.539148) picked at (17.768839, -2.539148) picked at (-18.088769, -2.539143) picked at (18.088769, -2.539143) picked at (-22.598153, -2.094669) picked at (22.59815, -2.094669) picked at (-24.866667, -1.983333) picked at (24.733332, -1.983333) picked at (25.489999, 12.1) picked at (25.393333, 12.416666) picked at (-25.490001, -1.766667) picked at (-25.393333, 12.383333) picked at (-25.490001, 12.1) picked at (25.489999, -1.766667) picked at (25.726667, 5.483333) picked at (25.489999, 12.7) picked at (-25.726667, 5.516666) picked at (-25.490001, 19) picked at (25.489999, -1.1) picked at (25.393333, 19.316666) picked at (25.399998, 8.116666) picked at (-25.636668, -2.25) picked at (-25.726667, -1.383334) picked at (-25.490001, -1.1) picked at (-25.393333, 19.283333) picked at (-25.400002, 8.116666) picked at (25.636665, -2.25) picked at (25.393333, -1.383334) picked at (25.489999, 19.6) picked at (25.399998, 16.683333) picked at (25.873333, 8.116666) picked at (-25.873334, -2.45) picked at (-25.490001, 19.6) picked at (-25.400002, 15.016666) picked at (-25.873334, 9.783333) picked at (25.686665, -2.45) picked at (25.399998, 1.216666) picked at (25.873333, 15.016666) picked at (-25.400002, 1.216666) picked at (-25.873334, 16.683333) picked at (25.686665, 2.883333) picked at (22.473627, 22.229735) picked at (25.399998, 21) picked at (-25.873334, 2.883333) picked at (-22.806963, 22.229735) picked at (-25.400002, 21) picked at (17.917968, 22.326792) picked at (25.873333, 21.05) picked at (-18.917967, 22.326792) picked at (-25.873334, 21.85) picked at (16.918149, 21.76373) picked at (14.082033, 22.326792) picked at (6.082593, 22.476137) picked at (-17.918148, 21.76373) picked at (-6.415925, 22.476137) picked at (-15.082032, 22.326792) picked at (15.793173, 22.25812) picked at (15.081852, 21.76373) picked at (1.917968, 22.326792) picked at (-16.76103, 22.289882) picked at (-16.081851, 21.76373) picked at (-1.917967, 22.326792) picked at (0.918149, 21.76373) picked at (-0.918148, 21.76373) picked at (0.269322, 21.884696) makes body 24
sketch "Sketch10" plane through (-26.06, 0, 0) normal (-1, 0, 0) x (0, -1, 0)
  line L0 (0, -22.65) -> (0, 2.65)
  line L1 (0, 2.65) -> (-12, 2.65)
  line L2 (-12, 2.65) -> (-12, -22.65)
  line L3 (-12, -22.65) -> (0, -22.65)
  arc A0 (-2, -3) -> (-1.998332, -16.999999) centre (-2.00417, -10) ccw
  line L4 (-2, -3) -> (-1.998332, -16.999999)
extrude "Extrude41" cut sketch "Sketch10" against normal blind 1 contours A0 L4 picked at (-4.629901, -7.66698) bodies 6 24
move_body "Move2" bodies 19 20 22 21 23 to x (1, 0, 0) y (0, 1, 0) z (0, 0, 1) at (3, 0, 0)
copy_body "CopyPasteBodies2" bodies 19 20 21 22 23 makes body 25 makes body 26 makes body 27 makes body 28 makes body 29
move_body "Move3" bodies 25 26 27 28 29 to x (1, 0, 0) y (0, 1, 0) z (0, 0, 1) at (0, 0, -70)
copy_body "CopyPasteBodies3" bodies 25 26 27 28 29 makes body 30 makes body 31 makes body 32 makes body 33 makes body 34
move_body "Move4" bodies 30 31 32 33 34 to x (1, 0, 0) y (0, 1, 0) z (0, 0, 1) at (56, 0, 0)
extrude "Extrude42" cut sketch "Blueprint" along normal blind 2 contours A6 picked at (-1.581142, 47.433122) bodies 6
extrude "Extrude43" cut sketch "Blueprint" along normal blind 2 contours A1 | A13 | A23 picked at (-28.447805, -34.584499) picked at (-26.11169, -34.534513) picked at (-29.306987, -35.12917) bodies 6
extrude "Extrude44" cut sketch "Blueprint" along normal blind 2 contours A3 | A15 | A21 picked at (27.665869, 35.49322) picked at (29.802492, 35.730779) picked at (27.55602, 33.763856) bodies 6
extrude "Extrude45" cut sketch "Blueprint" along normal blind 2 contours A4 | A14 | A22 picked at (-28.447805, 35.415501) picked at (-26.063404, 34.821149) picked at (-29.306987, 34.87083) bodies 6
extrude "Extrude46" cut sketch "Blueprint" along normal blind 2 from surface at 48 contours A0 L454 | A0 L40 L46 L454 | A0 L32 L40 L46 | A0 L32 L38 | A0 L38 L48 | A0 L42 L48 | A0 L42 picked at (-0.080266, 16.579553) picked at (-3, 10.157626) picked at (5.417667, 1.4) picked at (-5.900918, -1.983333) picked at (-5.882271, -2.766667) picked at (5.683555, -5.514289) picked at (-1.266033, -11.46973) bodies 14
extrude "Extrude47" add sketch "Blueprint" against normal blind 3.5 from surface at 48 contours L31 L32 L37 L38 L41 L47 L396 L399 L400 | L31 L32 L41 L47 L400 | A18 | A19 picked at (-25.490001, -1.766667) picked at (-25.02, -1.583333) picked at (39.611389, -23.686242) picked at (37.680599, -25.819207) bodies 14
extrude "Extrude48" add sketch "Blueprint" along normal blind 1 from surface at 43 separate body contours A0 L32 L40 L46 A46 | A0 L32 L40 L46 | A0 L32 L40 L46 A46 | L32 A16 L40 L46 A46 | A0 L32 L38 | A0 L32 L38 A46 | L32 A16 L40 L46 A46 | A0 L32 L38 A46 | L32 A16 L40 L43 L46 L49 L459 L462 L479 L480 L481 L484 L485 L489 L490 | A0 L38 L48 | A0 L38 L48 A46 | L32 L38 A16 A46 | L32 A16 L40 L41 L46 L47 L397 L400 L401 L407 L408 L411 L415 L416 L423 | A0 L38 L48 A46 | L32 L38 A16 A46 | L40 L43 L46 L49 L489 L490 | L38 A16 L48 A46 | L32 L38 A16 L397 | L40 L41 L46 L47 L416 L423 | L38 A16 L48 A46 | L32 L38 A16 L462 | L38 A16 L48 L397 | L32 L38 L41 L47 L397 | L32 L41 L47 L397 L400 | L38 A16 L48 L462 | L32 L43 L49 L459 L462 | L32 L38 L43 L49 L462 | L38 L41 L47 L48 L397 | L38 L43 L48 L49 L462 | L43 L49 L479 L480 L481 L484 L485 | L41 L47 L401 L407 L408 L411 L415 picked at (16.610892, 6.696031) picked at (5.417667, 1.4) picked at (-16.588449, 6.769971) picked at (16.955543, 6.695503) picked at (-5.900918, -1.983333) picked at (-17.768839, -2.539148) picked at (-16.933326, 6.769391) picked at (17.768839, -2.539148) picked at (22.633332, 0.538942) picked at (-5.882271, -2.766667) picked at (-17.703996, -2.961152) picked at (-18.088769, -2.539143) picked at (-22.551552, 3.200808) picked at (17.703996, -2.961152) picked at (18.088769, -2.539143) picked at (24.733332, 6.85) picked at (-18.061761, -2.727855) picked at (-22.598153, -2.094669) picked at (-24.866667, 6.85) picked at (18.061761, -2.727855) picked at (22.59815, -2.094669) picked at (-22.570428, -2.766667) picked at (-24.866667, -1.983333) picked at (-24.733335, -1.583333) picked at (22.570425, -2.766667) picked at (24.733332, -1.516667) picked at (24.733332, -1.983333) picked at (-24.866667, -2.766667) picked at (24.866666, -2.883333) picked at (24.866666, 2.355609) picked at (-24.866667, 1.744392) makes body 35
extrude "Extrude51" add sketch "Blueprint" along normal blind 37 separate body contours A15 picked at (29.802492, 35.730779) makes body 36
extrude "Extrude52" add sketch "Blueprint" along normal blind 37 separate body contours A10 | A11 picked at (26.387387, -34.993527) picked at (26.938574, -33.213382) makes body 37
extrude "Extrude53" add sketch "Blueprint" along normal blind 37 separate body contours A13 | A23 picked at (-26.11169, -34.534513) picked at (-29.306987, -35.12917) makes body 38
extrude "Extrude54" add sketch "Blueprint" along normal blind 37 separate body contours A14 | A22 picked at (-26.063404, 34.821149) picked at (-29.306987, 34.87083) makes body 39
extrude "Extrude56" cut 1 faces at (39.533614, 44.5, 23.714429) along direction (0, 1, 0) blind 3.5 on bodies 14 bodies 14
extrude "Extrude57" cut 1 faces at (-25.470001, 44.5, 1.7) along direction (0, 1, 0) blind 3.5 on bodies 14 bodies 14
extrude "Extrude59" add sketch "Sketch8" against normal blind 1.8 contours A7 A8 L1 L2 L166 | A7 A8 L166 L167 | A7 A8 L167 L173 | A7 A8 L3 L170 | A7 A8 L170 L173 picked at (10.419576, -14.962984) picked at (11.812408, 13.909637) picked at (-8.241935, 16.262679) picked at (-15.610505, -9.429752) picked at (-12.96051, 13.151425) bodies 14
extrude "Extrude60" add sketch "Sketch8" against normal blind 3.5 contours A9 | A14 | A15 | A18 | A21 | A24 | A27 | A30 | A33 | A36 | A39 picked at (-14.046923, 17.368666) picked at (-14.046923, 25.368666) picked at (18.953077, 25.368666) picked at (18.953077, 17.368666) picked at (40.611389, 27.41376) picked at (40.611389, -20.88624) picked at (18.953077, -22.931334) picked at (1.953077, -22.931334) picked at (-14.046923, -22.931334) picked at (-38.388611, -20.88624) picked at (-38.388611, 27.41376) bodies 14
extrude "Extrude61" add sketch "Sketch8" against normal blind 1.1 separate body contours L8 L9 L10 L11 | L12 L13 L17 L19 | L20 L21 L23 L28 | L29 L30 L33 L36 | L37 L38 L42 L43 L44 L45 L46 L47 | L48 L49 L53 L57 | L55 L58 L59 L64 | L63 L65 L66 L71 picked at (-28.883331, 22.4) picked at (-28.883331, 15.5) picked at (-28.883331, 14.9) picked at (-28.883331, 8) picked at (-30.899998, -1.744392) picked at (-28.883331, -12.1) picked at (-28.883331, -12.7) picked at (-24.849998, -21.866666) makes body 40 at (28.883331, 48, -12.1) makes body 41 at (28.883331, 48, 22.4) makes body 42 at (28.883331, 48, 15.5) makes body 43 at (28.883331, 48, -12.7) makes body 44 at (28.883331, 48, 8) makes body 45 at (28.883331, 48, 1.1) makes body 46 at (28.883331, 48, 14.9) makes body 47 at (24.849998, 48, -21.866666)